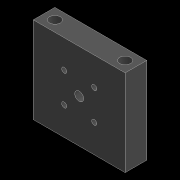
# Autodesk Inventor part: MotorMounts
Saved by Autodesk Inventor 2022 (Build 260153000, 153)
## iProperties
Created: 2022-09-20
Part Number: MotorMounts
Material: Custom TPU
Document SubType Name: Modeling
Designer: tandu
Density: 1.21 g/cm^3
Appearance: Generic
Author: tandu
Autodesk Inventor part; units mm, degrees
ref_plane "YZ Plane" through (0, 0, 0) normal (1, 0, 0) x (0, 1, 0)
ref_plane "XZ Plane" through (0, 0, 0) normal (0, 1, 0) x (-1, 0, 0)
ref_plane "XY Plane" through (0, 0, 0) normal (0, 0, 1) x (1, 0, 0)
sketch "Sketch1" plane through (0, 0, 0) normal (0, 0, 1) x (1, 0, 0)
  circle A0 centre (0, 0) radius 12.5 construction
  circle A1 centre (8.8388, 8.8388) radius 1.5
  circle A2 centre (-8.8388, 8.8388) radius 1.5
  circle A3 centre (-8.8388, -8.8388) radius 1.5
  circle A4 centre (8.8388, -8.8388) radius 1.5
  circle A5 centre (0, 0) radius 3.627
  circle A6 centre (0, 0) radius 2.627
  line L0 (-27.025, -25.4) -> (27.025, -25.4)
  line L1 (27.025, -25.4) -> (27.025, 25.4)
  line L2 (27.025, 25.4) -> (-27.025, 25.4)
  line L3 (-27.025, 25.4) -> (-27.025, -25.4)
  line L4 (-27.025, -25.4) -> (27.025, 25.4) construction
  line L5 (27.025, -25.4) -> (-27.025, 25.4) construction
  dimension "d0" = 25
  dimension "d1" = 3
  dimension "d4" = 360
  dimension "d6" = 7.254
  dimension "d7" = 5.254
  dimension "d8" = 54.05
  dimension "d9" = 50.8
  constraints: 12 end point, 6 centre point, 3 coincident, 2 midpoint, 2 parallel, 1 horizontal, 1 horizontal alignment, 1 perpendicular, 12 other
  measures "d1" diameter of A1
  measures "d6" diameter of A5
  measures "d7" diameter of A6
  measures "d8" distance of L2.end L1.end
  measures "d9" distance of L0.end L1.end
extrude "BaseExtrusion" add sketch "Sketch1" against normal blind 12.7 contours A5 | L3 L2 L1 L0
sketch "Sketch3" plane through (0, 0, -12.7) normal (0, 0, -1) x (-1, 0, 0)
  circle A0 centre (0, 0) radius 18.135
  circle A1 centre (0, 0) radius 3.5
  circle A2 centre (0, 0) radius 2.5
  circle A3 centre (0, 0) radius 12.5 construction
  circle A4 centre (8.8388, -8.8388) radius 1.5
  circle A5 centre (-8.8388, -8.8388) radius 1.5
  circle A6 centre (-8.8388, 8.8388) radius 1.5
  circle A7 centre (8.8388, 8.8388) radius 1.5
  line L0 (-8.8388, 8.8388) -> (8.8388, -8.8388) construction
  line L1 (-8.8388, -8.8388) -> (8.8388, 8.8388) construction
  circle A8 centre (-8.8388, -8.8388) radius 3.3175 construction
  circle A9 centre (8.8388, -8.8388) radius 3.3175 construction
  circle A10 centre (8.8388, 8.8388) radius 3.3175 construction
  circle A11 centre (-8.8388, 8.8388) radius 3.3175 construction
  arc A12 (-10.3798, 14.8707) -> (10.3798, 14.8707) centre (0, 22.2158) ccw
  arc A13 (-14.8707, -10.3798) -> (-14.8707, 10.3798) centre (-22.2158, 0) ccw
  arc A14 (14.8707, 10.3798) -> (14.8707, -10.3798) centre (22.2158, 0) ccw
  dimension "d17" = 36.27
  dimension "d18" = 7
  dimension "d19" = 5
  dimension "d20" = 25
  dimension "d21" = 3
  dimension "d22" = 6.6351
  dimension "d23" = 12.7158
  constraints: 16 point on circle, 15 centre point, 8 coincident, 8 equal radius, 6 tangent, 4 end point, 4 midpoint, 1 horizontal alignment, 1 perpendicular
  measures "d17" diameter of A0
  measures "d18" diameter of A1
  measures "d19" diameter of A2
  measures "d20" diameter of A3
  measures "d21" diameter of A4
  measures "d22" diameter of A8
  measures "d23" radius of A14
extrude "Extrusion4" cut sketch "Sketch3" against normal blind 6.4 contours A14 A0 A13 A12 | A1
extrude "MotorNubSlot" cut sketch "Sketch1" along normal blind 1.2 from surface at -6.3 contours A5
sketch "Sketch2" plane through (-27.025, 25.4, 0) normal (0, 1, 0) x (1, 0, 0)
  line L0 (54.05, 0) -> (0, 0) projected
  line L1 (54.05, 0) -> (54.05, 12.7) projected
  line L2 (0, 12.7) -> (54.05, 12.7) projected
  line L3 (0, 0) -> (0, 12.7) projected
  circle A0 centre (6.35, 6.35) radius 6.35 construction
  circle A1 centre (47.7, 6.35) radius 6.35 construction
  circle A2 centre (6.35, 6.35) radius 3.175
  circle A3 centre (47.7, 6.35) radius 3.175
  point P0 (27.025, 0)
  dimension "d14" = 6.35
  constraints: 6 tangent, 4 centre point, 2 coincident, 1 equal radius
  measures "d14" diameter of A2
extrude "Standoff Holes" cut sketch "Sketch2" against normal through all contours A2 | A3
equation "\"d8\" = MotorMountWidth"
equation "\"d9\" = MotorMountHeight"
equation "\"d10\" = MotorMountThickness"
equation "\"MotorMountHeight\" = StandOffHeight - 2 * AluminumBottomThickness - 2 * TPUBottomThickness"
equation "\"MotorMountWidth\" = 54.05"
equation "\"MotorMountThickness\" = 12.7"
equation "\"StandOffHeight\" = 57.15"
equation "\"AluminumBottomThickness\" = 1.5875"
equation "\"TPUBottomThickness\" = 1.5875"
body "Solid1"
